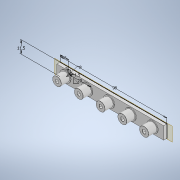
# Autodesk Inventor part: insert_testing_3Dprint
Saved by Autodesk Inventor 2021 (Build 250183000, 183)
## iProperties
Created: 2021-08-12
Part Number: insert_testing_3Dprint
Material: Generic
Document SubType Name: Modeling
Designer: fu18427
Density: 1 g/cm^3
Appearance: Default
Author: fu18427
Autodesk Inventor part; units mm, degrees
ref_plane "YZ Plane" through (0, 0, 0) normal (1, 0, 0) x (0, 1, 0)
ref_plane "XZ Plane" through (0, 0, 0) normal (0, 1, 0) x (-1, 0, 0)
sketch "Sketch1" plane through (0, 0, 0) normal (0, 0, 1) x (1, 0, 0)
  line L0 (0, 0) -> (98, 0)
  line L1 (98, 0) -> (98, 11.5)
  line L2 (98, 11.5) -> (0, 11.5)
  line L3 (0, 11.5) -> (0, 0)
  circle A0 centre (8, 5.75) radius 4
  arc A1 (7, 4.632) -> (7, 6.868) centre (8, 5.75) ccw
  line L4 (7, 6.868) -> (7, 4.632)
  circle A2 centre (28, 5.75) radius 4
  arc A3 (27, 4.632) -> (27, 6.868) centre (28, 5.75) ccw
  line L5 (27, 6.868) -> (27, 4.632)
  circle A4 centre (48, 5.75) radius 4
  arc A5 (47, 4.632) -> (47, 6.868) centre (48, 5.75) ccw
  line L6 (47, 6.868) -> (47, 4.632)
  circle A6 centre (68, 5.75) radius 4
  arc A7 (67, 4.632) -> (67, 6.868) centre (68, 5.75) ccw
  line L7 (67, 6.868) -> (67, 4.632)
  circle A8 centre (88, 5.75) radius 4
  arc A9 (87, 4.632) -> (87, 6.868) centre (88, 5.75) ccw
  line L8 (87, 6.868) -> (87, 4.632)
  point P0 (0, 5.75)
  dimension "d0" = 11.5
  dimension "d1" = 8
  dimension "d2" = 8
  dimension "d3" = 1.5
  dimension "d4" = 1
  dimension "d7" = 20
  dimension "d12" = 98
  constraints: 18 end point, 10 centre point, 10 point on circle, 5 coincident, 2 horizontal, 2 parallel, 1 horizontal alignment, 1 midpoint, 1 perpendicular, 1 vertical, 28 other
  measures "d0" distance of L2.end L0.start
  measures "d1" diameter of A0
  measures "d2" distance from line of L3 A0.centre
  measures "d3" radius of A1
  measures "d4" distance from line of L4 A0.centre
  measures "d7" distance of A0.centre A2.centre
  measures "d12" distance of L1.end L2.end
extrude "Extrusion1" add sketch "Sketch1" along normal blind 3 contours L3 L2 L1 L0 | A0 | L4 A1 | A2 | L5 A3 | A4 | L6 A5 | A6 | L7 A7 | A8 | L8 A9
sketch "Sketch2" plane through (0, 0, 3) normal (0, 0, 1) x (1, 0, 0)
  circle A0 centre (8, 5.75) radius 4 projected
  arc A1 (7, 4.632) -> (7, 6.868) centre (8, 5.75) ccw projected
  line L0 (7, 6.868) -> (7, 4.632) projected
  circle A2 centre (28, 5.75) radius 4 construction
  arc A3 (27, 4.632) -> (27, 6.868) centre (28, 5.75) ccw construction
  line L1 (27, 6.868) -> (27, 4.632) construction
  line L2 (47, 6.868) -> (47, 4.632) construction
  arc A4 (47, 4.632) -> (47, 6.868) centre (48, 5.75) ccw construction
  circle A5 centre (48, 5.75) radius 4 construction
  circle A6 centre (68, 5.75) radius 4 construction
  arc A7 (67, 4.632) -> (67, 6.868) centre (68, 5.75) ccw construction
  line L3 (67, 6.868) -> (67, 4.632) construction
  line L4 (87, 6.868) -> (87, 4.632) construction
  arc A8 (87, 4.632) -> (87, 6.868) centre (88, 5.75) ccw construction
  circle A9 centre (88, 5.75) radius 4 construction
  circle A10 centre (28, 5.75) radius 4.05
  arc A11 (26.95, 4.6098) -> (26.95, 6.8902) centre (28, 5.75) ccw
  line L5 (26.95, 4.6098) -> (26.95, 6.8902)
  circle A12 centre (48, 5.75) radius 4.1
  line L6 (46.9, 4.5881) -> (46.9, 6.9119)
  arc A13 (46.9, 4.5881) -> (46.9, 6.9119) centre (48, 5.75) ccw
  circle A14 centre (68, 5.75) radius 4.15
  arc A15 (66.85, 4.5668) -> (66.85, 6.9332) centre (68, 5.75) ccw
  line L7 (66.85, 4.5668) -> (66.85, 6.9332)
  line L8 (86.8, 4.5458) -> (86.8, 6.9542)
  arc A16 (86.8, 4.5458) -> (86.8, 6.9542) centre (88, 5.75) ccw
  circle A17 centre (88, 5.75) radius 4.2
  point P0 (0, 0)
  dimension "d15" = 0.05
  dimension "d17" = 0.05
  dimension "d18" = 0.1
  dimension "d19" = 0.1
  dimension "d20" = 0.15
  dimension "d21" = 0.15
  dimension "d22" = 0.2
  dimension "d23" = 0.2
  constraints: 8 centre point, 8 end point, 8 point on circle, 4 other
  measures "d15" radial gap between concentric circles of A10 A2
  measures "d17" radial gap between concentric circles of A3 A11
  measures "d18" radial gap between concentric circles of A5 A12
  measures "d19" radial gap between concentric circles of A4 A13
  measures "d20" radial gap between concentric circles of A6 A14
  measures "d21" radial gap between concentric circles of A7 A15
  measures "d22" radial gap between concentric circles of A9 A17
  measures "d23" radial gap between concentric circles of A8 A16
extrude "Extrusion2" add sketch "Sketch2" along normal blind 8
sketch "Sketch3" plane through (0, 0, 3) normal (0, 0, 1) x (1, 0, 0)
  circle A0 centre (8, 5.75) radius 4 projected
  circle A1 centre (8, 5.75) radius 5
  line L0 (0, 0) -> (98, 0) projected
  circle A2 centre (28, 5.75) radius 5
  circle A3 centre (48, 5.75) radius 5
  circle A4 centre (68, 5.75) radius 5
  circle A5 centre (88, 5.75) radius 5
  dimension "d26" = 1
  dimension "d29" = 20
  constraints: 5 centre point, 1 horizontal, 8 other
  measures "d26" radial gap between concentric circles of A0 A1
  measures "d29" distance of A0.centre A2.centre
extrude "Extrusion3" add sketch "Sketch3" along normal blind 0.5 contours A0 | A1 | A2 | A3 | A4 | A5
chamfer "Chamfer1" distance 0.1 angle 45 15 edges at (4, 5.75, 11) (9.5, 5.75, 11) (7, 5.75, 11) (23.95, 5.75, 11) (29.55, 5.75, 11) (26.95, 5.75, 11) (43.9, 5.75, 11) (49.6, 5.75, 11) (46.9, 5.75, 11) (69.65, 5.75, 11) (66.85, 5.75, 11) (63.85, 5.75, 11) (83.8, 5.75, 11) (89.7, 5.75, 11) (86.8, 5.75, 11)
sketch "Sketch4" plane through (0, 0, 3) normal (0, 0, 1) x (1, 0, 0)
  line L0 (15, 8.25) -> (15, 3.25)
  line L1 (15, 3.25) -> (20, 5.75)
  line L2 (20, 5.75) -> (15, 8.25)
  line L3 (0, 11.5) -> (0, 0) projected
  line L4 (0, 5.75) -> (37.8806, 5.75)
  dimension "d39" = 15
  dimension "d40" = 5
  dimension "d41" = 5
  constraints: 8 end point, 1 horizontal, 1 midpoint, 1 vertical, 1 other
  measures "d39" distance between parallel lines of L3 L0
  measures "d40" distance from line of L0 L1.end
  measures "d41" distance of L0.start L0.end
extrude "Extrusion4" cut sketch "Sketch4" against normal blind 0.5
body "Solid1"
